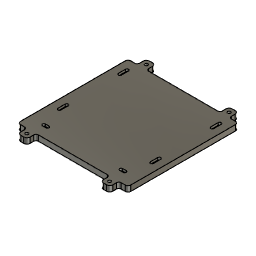
base_mount (Autodesk Fusion 360 design; units mm, degrees)
Autodesk Fusion 360 part; units mm, degrees
sketch "Sketch1" plane through (0, 0, 0) normal (0, 0, 1) x (1, 0, 0)
  line L0 (60, -60) -> (-60, -60)
  line L1 (-60, -60) -> (-60, 60)
  line L2 (-60, 60) -> (60, 60)
  line L3 (60, 60) -> (60, -60)
  line L4 (60, -60) -> (-60, 60) construction
  line L5 (-60, -60) -> (60, 60) construction
  dimension "d4" = 120
  dimension "d5" = 120
  constraint perpendicular L0 L1
  constraint parallel L0 L2
  constraint parallel L1 L3
  constraint horizontal L0
  constraint coincident L4 origin
  constraint coincident L5 origin
  measures "d4" distance of L1.end L2.end
  measures "d5" distance of L0.end L1.end
extrude "Extrude1" add sketch "Sketch1" along normal blind 6
sketch "Sketch2" plane through (0, 0, 0) normal (0, 0, -1) x (1, 0, 0)
  line L0 (-60, -60) -> (60, -60)
  line L1 (60, -60) -> (60, 60)
  line L2 (60, 60) -> (-60, 60)
  line L3 (-60, 60) -> (-60, -60)
  line L4 (-44, 44.625) -> (-40, 44.625)
  arc A0 (-40, 44.625) -> (-40, 50.375) centre (-40, 47.5) ccw
  line L5 (-40, 50.375) -> (-44, 50.375)
  arc A1 (-44, 50.375) -> (-44, 44.625) centre (-44, 47.5) ccw
  line L6 (-44, 47.5) -> (-40, 47.5) construction
  point P0 (-42, 47.5)
  dimension "d14" = 5.75
  dimension "d15" = 4
  dimension "d16" = 12.5
  dimension "d17" = 18
  constraint tangent L4 A0
  constraint tangent A0 L5
  constraint parallel L4 L5
  constraint tangent L5 A1
  constraint tangent L4 A1
  constraint horizontal L6
  constraint midpoint L6 P0
  measures "d14" diameter of A0
  measures "d15" distance of A1.centre A0.centre
  measures "d16" distance of L2 P0
  measures "d17" distance of L3 P0
extrude "Extrude2" cut sketch "Sketch2" against normal blind 3.5 contours L4 A0 L5 A1
sketch "Sketch3" plane through (0, 0, 3.5) normal (0, 0, -1) x (1, 0, 0)
  arc A0 (-44, 50.375) -> (-44, 44.625) centre (-44, 47.5) ccw
  line L0 (-44, 44.625) -> (-40, 44.625)
  arc A1 (-40, 44.625) -> (-40, 50.375) centre (-40, 47.5) ccw
  line L1 (-40, 50.375) -> (-44, 50.375)
  line L2 (-44, 45.875) -> (-40, 45.875)
  arc A2 (-40, 45.875) -> (-40, 49.125) centre (-40, 47.5) ccw
  line L3 (-40, 49.125) -> (-44, 49.125)
  arc A3 (-44, 49.125) -> (-44, 45.875) centre (-44, 47.5) ccw
  line L4 (-44, 47.5) -> (-40, 47.5) construction
  line L5 (60, 60) -> (-60, 60)
  line L6 (-60, 60) -> (-60, -60)
  point P0 (-42, 47.5)
  dimension "d20" = 3.25
  dimension "d21" = 4
  dimension "d22" = 12.5
  dimension "d23" = 18
  constraint tangent L2 A2
  constraint tangent A2 L3
  constraint parallel L2 L3
  constraint tangent L3 A3
  constraint tangent L2 A3
  constraint parallel L0 L4
  constraint midpoint L4 P0
  measures "d20" diameter of A2
  measures "d21" distance of A0.centre A1.centre
  measures "d22" distance of P0 L5
  measures "d23" distance of P0 L6
extrude "Extrude3" cut sketch "Sketch3" against normal up to surface (2.5 mm away) contours L2 A2 L3 A3
mirror "Mirror1" about plane through (0, 0, 0) normal (1, 0, 0) of "Extrude2", "Extrude3"
sketch "Sketch4" plane through (0, 0, 0) normal (0, 0, -1) x (1, 0, 0)
  line L0 (44, 44.625) -> (40, 44.625)
  arc A0 (40, 50.375) -> (40, 44.625) centre (40, 47.5) ccw
  line L1 (40, 50.375) -> (44, 50.375)
  arc A1 (44, 44.625) -> (44, 50.375) centre (44, 47.5) ccw
  line L2 (-40, 44.625) -> (-44, 44.625)
  arc A2 (-44, 50.375) -> (-44, 44.625) centre (-44, 47.5) ccw
  line L3 (-44, 50.375) -> (-40, 50.375)
  arc A3 (-40, 44.625) -> (-40, 50.375) centre (-40, 47.5) ccw
  line L4 (-60, -60) -> (60, -60)
  line L5 (60, -60) -> (60, 60)
  line L6 (60, 60) -> (-60, 60)
  line L7 (-60, 60) -> (-60, -60)
  line L8 (60, -60) -> (-60, -60) construction
  line L9 (-60, -60) -> (-60, 35) construction
  line L10 (-60, 35) -> (60, 35) construction
  line L11 (60, 35) -> (60, -60) construction
  line L12 (0, 35) -> (0, -60) construction
  line L13 (60, -12.5) -> (-60, -12.5) construction
  line L14 (-50.35, -45.35) -> (50.35, -45.35) construction
  line L15 (50.35, -45.35) -> (50.35, 20.35) construction
  line L16 (50.35, 20.35) -> (-50.35, 20.35) construction
  line L17 (-50.35, 20.35) -> (-50.35, -45.35) construction
  line L18 (-50.35, -45.35) -> (50.35, 20.35) construction
  line L19 (50.35, -45.35) -> (-50.35, 20.35) construction
  line L20 (47.475, 24.35) -> (47.475, 16.35)
  arc A4 (47.475, 16.35) -> (53.225, 16.35) centre (50.35, 16.35) ccw
  line L21 (53.225, 16.35) -> (53.225, 24.35)
  arc A5 (53.225, 24.35) -> (47.475, 24.35) centre (50.35, 24.35) ccw
  line L22 (50.35, 24.35) -> (50.35, 16.35) construction
  line L23 (51.975, 16.35) -> (51.975, 24.35)
  arc A6 (51.975, 24.35) -> (48.725, 24.35) centre (50.35, 24.35) ccw
  line L24 (48.725, 24.35) -> (48.725, 16.35)
  arc A7 (48.725, 16.35) -> (51.975, 16.35) centre (50.35, 16.35) ccw
  line L25 (50.35, 16.35) -> (50.35, 24.35) construction
  point P0 (0, -12.5)
  point P1 (50.35, 20.35)
  point P2 (50.35, 20.35)
  dimension "d29" = 95
  dimension "d30" = 65.7
  dimension "d31" = 100.7
  dimension "d36" = 5.75
  dimension "d37" = 8
  dimension "d38" = 3.25
  dimension "d39" = 8
  constraint horizontal L8
  constraint vertical L9
  constraint horizontal L10
  constraint vertical L11
  constraint coincident L4.end L5.start
  constraint midpoint L10 L12.start
  constraint midpoint L8 L12.end
  constraint midpoint L11 L13.start
  constraint midpoint L9 L13.end
  constraint perpendicular L14 L15
  constraint parallel L14 L16
  constraint parallel L15 L17
  constraint horizontal L14
  constraint coincident L18 P0
  constraint coincident L19 P0
  constraint midpoint L13 P0
  constraint tangent L20 A4
  constraint tangent A4 L21
  constraint parallel L20 L21
  constraint tangent L21 A5
  constraint tangent L20 A5
  constraint coincident L15 A4.centre
  constraint perpendicular L16 L22
  constraint coincident P2 P1
  constraint midpoint L22 P2
  constraint tangent L23 A6
  constraint tangent A6 L24
  constraint parallel L23 L24
  constraint tangent L24 A7
  constraint tangent L23 A7
  constraint coincident L22 A5.centre
  constraint perpendicular L16 L25
  constraint midpoint L25 P2
  measures "d29" distance of L4.end L10.end
  measures "d30" distance of L14.end P2
  measures "d31" distance of P2 L16.end
  measures "d36" diameter of A4
  measures "d37" distance of A5.centre A4.centre
  measures "d38" diameter of A6
  measures "d39" distance of A4.centre A5.centre
extrude "Extrude4" cut sketch "Sketch4" against normal blind 3.5 contours L20 A4 L21 A5
extrude "Extrude5" cut sketch "Sketch4" against normal up to surface (6 mm away) contours L23 A6 L24 A7
pattern_linear "R-Pattern1" count 2 spacing 100.7 along (-1, 0, 0) count 2 spacing 65.7 along (0, 1, 0) of "Extrude4", "Extrude5"
sketch "Sketch5" plane through (0, 0, 0) normal (0, 0, -1) x (1, 0, 0)
  line L0 (47.475, -49.35) -> (47.475, -41.35)
  arc A0 (53.225, -41.35) -> (47.475, -41.35) centre (50.35, -41.35) ccw
  line L1 (53.225, -41.35) -> (53.225, -49.35)
  arc A1 (47.475, -49.35) -> (53.225, -49.35) centre (50.35, -49.35) ccw
  line L2 (47.475, 16.35) -> (47.475, 24.35)
  arc A2 (53.225, 24.35) -> (47.475, 24.35) centre (50.35, 24.35) ccw
  line L3 (53.225, 24.35) -> (53.225, 16.35)
  arc A3 (47.475, 16.35) -> (53.225, 16.35) centre (50.35, 16.35) ccw
  line L4 (44, 44.625) -> (40, 44.625)
  arc A4 (40, 50.375) -> (40, 44.625) centre (40, 47.5) ccw
  line L5 (40, 50.375) -> (44, 50.375)
  arc A5 (44, 44.625) -> (44, 50.375) centre (44, 47.5) ccw
  line L6 (-40, 44.625) -> (-44, 44.625)
  arc A6 (-44, 50.375) -> (-44, 44.625) centre (-44, 47.5) ccw
  line L7 (-44, 50.375) -> (-40, 50.375)
  arc A7 (-40, 44.625) -> (-40, 50.375) centre (-40, 47.5) ccw
  line L8 (-60, -60) -> (60, -60)
  line L9 (60, -60) -> (60, 60)
  line L10 (60, 60) -> (-60, 60)
  line L11 (-60, 60) -> (-60, -60)
  line L12 (-53.225, 16.35) -> (-53.225, 24.35)
  arc A8 (-47.475, 24.35) -> (-53.225, 24.35) centre (-50.35, 24.35) ccw
  line L13 (-47.475, 24.35) -> (-47.475, 16.35)
  arc A9 (-53.225, 16.35) -> (-47.475, 16.35) centre (-50.35, 16.35) ccw
  line L14 (-53.225, -49.35) -> (-53.225, -41.35)
  arc A10 (-47.475, -41.35) -> (-53.225, -41.35) centre (-50.35, -41.35) ccw
  line L15 (-47.475, -41.35) -> (-47.475, -49.35)
  arc A11 (-53.225, -49.35) -> (-47.475, -49.35) centre (-50.35, -49.35) ccw
  line L16 (49.25, 50) -> (-49.25, 50) construction
  line L17 (-49.25, 50) -> (-49.25, -50) construction
  line L18 (-49.25, -50) -> (49.25, -50) construction
  line L19 (49.25, -50) -> (49.25, 50) construction
  line L20 (49.25, 50) -> (-49.25, -50) construction
  line L21 (-49.25, 50) -> (49.25, -50) construction
  line L22 (7.5, 50.4) -> (-2.5, 50.4)
  line L23 (-2.5, 50.4) -> (-2.5, 52.4)
  line L24 (-2.5, 52.4) -> (7.5, 52.4)
  line L25 (7.5, 52.4) -> (7.5, 50.4)
  line L26 (7.5, 50.4) -> (-2.5, 52.4) construction
  line L27 (-2.5, 50.4) -> (7.5, 52.4) construction
  line L28 (-51.65, 5.3028) -> (-49.65, 5.3028)
  line L29 (-49.65, 5.3028) -> (-49.65, -4.6972)
  line L30 (-49.65, -4.6972) -> (-51.65, -4.6972)
  line L31 (-51.65, -4.6972) -> (-51.65, 5.3028)
  line L32 (-51.65, 5.3028) -> (-49.65, -4.6972) construction
  line L33 (-49.65, 5.3028) -> (-51.65, -4.6972) construction
  line L34 (51.65, -5) -> (49.65, -5)
  line L35 (49.65, -5) -> (49.65, 5)
  line L36 (49.65, 5) -> (51.65, 5)
  line L37 (51.65, 5) -> (51.65, -5)
  line L38 (51.65, -5) -> (49.65, 5) construction
  line L39 (49.65, -5) -> (51.65, 5) construction
  line L40 (5.2107, -52.4) -> (-4.7893, -52.4)
  line L41 (-4.7893, -52.4) -> (-4.7893, -50.4)
  line L42 (-4.7893, -50.4) -> (5.2107, -50.4)
  line L43 (5.2107, -50.4) -> (5.2107, -52.4)
  line L44 (5.2107, -52.4) -> (-4.7893, -50.4) construction
  line L45 (-4.7893, -52.4) -> (5.2107, -50.4) construction
  point P0 (2.5, 51.4)
  point P1 (-50.65, 0.3028)
  point P2 (50.65, 0)
  point P3 (0.2107, -51.4)
  dimension "d50" = 100
  dimension "d51" = 98.5
  dimension "d56" = 10
  dimension "d57" = 2
  dimension "d58" = 0.4
  dimension "d59" = 10
  dimension "d60" = 2
  dimension "d61" = 0.4
  dimension "d62" = 2
  dimension "d63" = 10
  dimension "d64" = 0.4
  dimension "d65" = 10
  dimension "d66" = 2
  dimension "d67" = 0.4
  constraint perpendicular L16 L17
  constraint parallel L16 L18
  constraint parallel L17 L19
  constraint horizontal L16
  constraint coincident L20 origin
  constraint coincident L21 origin
  constraint perpendicular L22 L23
  constraint parallel L22 L24
  constraint parallel L23 L25
  constraint horizontal L22
  constraint coincident L26 P0
  constraint coincident L27 P0
  constraint perpendicular L28 L29
  constraint parallel L28 L30
  constraint parallel L29 L31
  constraint horizontal L28
  constraint coincident L32 P1
  constraint coincident L33 P1
  constraint perpendicular L34 L35
  constraint parallel L34 L36
  constraint parallel L35 L37
  constraint horizontal L34
  constraint coincident L38 P2
  constraint coincident L39 P2
  constraint perpendicular L40 L41
  constraint parallel L40 L42
  constraint parallel L41 L43
  constraint horizontal L40
  constraint coincident L44 P3
  constraint coincident L45 P3
  measures "d50" distance of L16.end L17.end
  measures "d51" distance of L17.end L18.end
  measures "d56" distance of L23.end L24.end
  measures "d57" distance of L22.end L23.end
  measures "d58" distance of L16 L22
  measures "d59" distance of L28.end L29.end
  measures "d60" distance of L29.end L30.end
  measures "d61" distance of L17 L29
  measures "d62" distance of L35.end L36.end
  measures "d63" distance of L34.end L35.end
  measures "d64" distance of L19 L35
  measures "d65" distance of L41.end L42.end
  measures "d66" distance of L40.end L41.end
  measures "d67" distance of L18 L42
extrude "Extrude6" add sketch "Sketch5" along normal blind 3.5 contours L22 L23 L24 L25 | L28 L29 L30 L31 | L34 L35 L36 L37 | L40 L41 L42 L43
sketch "Sketch6" plane through (0, 0, 6) normal (0, 0, 1) x (-1, 0, 0)
  line L0 (51.975, -41.35) -> (51.975, -49.35)
  arc A0 (48.725, -49.35) -> (51.975, -49.35) centre (50.35, -49.35) ccw
  line L1 (48.725, -49.35) -> (48.725, -41.35)
  arc A1 (51.975, -41.35) -> (48.725, -41.35) centre (50.35, -41.35) ccw
  line L2 (-48.725, -41.35) -> (-48.725, -49.35)
  arc A2 (-51.975, -49.35) -> (-48.725, -49.35) centre (-50.35, -49.35) ccw
  line L3 (-51.975, -49.35) -> (-51.975, -41.35)
  arc A3 (-48.725, -41.35) -> (-51.975, -41.35) centre (-50.35, -41.35) ccw
  line L4 (51.975, 24.35) -> (51.975, 16.35)
  arc A4 (48.725, 16.35) -> (51.975, 16.35) centre (50.35, 16.35) ccw
  line L5 (48.725, 16.35) -> (48.725, 24.35)
  arc A5 (51.975, 24.35) -> (48.725, 24.35) centre (50.35, 24.35) ccw
  line L6 (-48.725, 24.35) -> (-48.725, 16.35)
  arc A6 (-51.975, 16.35) -> (-48.725, 16.35) centre (-50.35, 16.35) ccw
  line L7 (-51.975, 16.35) -> (-51.975, 24.35)
  arc A7 (-48.725, 24.35) -> (-51.975, 24.35) centre (-50.35, 24.35) ccw
  line L8 (-40, 45.875) -> (-44, 45.875)
  arc A8 (-44, 49.125) -> (-44, 45.875) centre (-44, 47.5) ccw
  line L9 (-44, 49.125) -> (-40, 49.125)
  arc A9 (-40, 45.875) -> (-40, 49.125) centre (-40, 47.5) ccw
  line L10 (40, 49.125) -> (44, 49.125)
  arc A10 (44, 45.875) -> (44, 49.125) centre (44, 47.5) ccw
  line L11 (44, 45.875) -> (40, 45.875)
  arc A11 (40, 49.125) -> (40, 45.875) centre (40, 47.5) ccw
  line L12 (-60, -60) -> (60, -60)
  line L13 (60, -60) -> (60, 60)
  line L14 (60, 60) -> (-60, 60)
  line L15 (-60, 60) -> (-60, -60)
sketch "Sketch7" plane through (0, 0, 6) normal (0, 0, 1) x (-1, 0, 0)
  line L0 (51.975, -41.35) -> (51.975, -49.35)
  arc A0 (48.725, -49.35) -> (51.975, -49.35) centre (50.35, -49.35) ccw
  line L1 (48.725, -49.35) -> (48.725, -41.35)
  arc A1 (51.975, -41.35) -> (48.725, -41.35) centre (50.35, -41.35) ccw
  line L2 (-48.725, -41.35) -> (-48.725, -49.35)
  arc A2 (-51.975, -49.35) -> (-48.725, -49.35) centre (-50.35, -49.35) ccw
  line L3 (-51.975, -49.35) -> (-51.975, -41.35)
  arc A3 (-48.725, -41.35) -> (-51.975, -41.35) centre (-50.35, -41.35) ccw
  line L4 (51.975, 24.35) -> (51.975, 16.35)
  arc A4 (48.725, 16.35) -> (51.975, 16.35) centre (50.35, 16.35) ccw
  line L5 (48.725, 16.35) -> (48.725, 24.35)
  arc A5 (51.975, 24.35) -> (48.725, 24.35) centre (50.35, 24.35) ccw
  line L6 (-48.725, 24.35) -> (-48.725, 16.35)
  arc A6 (-51.975, 16.35) -> (-48.725, 16.35) centre (-50.35, 16.35) ccw
  line L7 (-51.975, 16.35) -> (-51.975, 24.35)
  arc A7 (-48.725, 24.35) -> (-51.975, 24.35) centre (-50.35, 24.35) ccw
  line L8 (-40, 45.875) -> (-44, 45.875)
  arc A8 (-44, 49.125) -> (-44, 45.875) centre (-44, 47.5) ccw
  line L9 (-44, 49.125) -> (-40, 49.125)
  arc A9 (-40, 45.875) -> (-40, 49.125) centre (-40, 47.5) ccw
  line L10 (40, 49.125) -> (44, 49.125)
  arc A10 (44, 45.875) -> (44, 49.125) centre (44, 47.5) ccw
  line L11 (44, 45.875) -> (40, 45.875)
  arc A11 (40, 49.125) -> (40, 45.875) centre (40, 47.5) ccw
  line L12 (-60, -60) -> (60, -60)
  line L13 (60, -60) -> (60, 60)
  line L14 (60, 60) -> (-60, 60)
  line L15 (-60, 60) -> (-60, -60)
  line L16 (50, 60) -> (40, 60)
  line L17 (40, 60) -> (40, 70)
  line L18 (40, 70) -> (50, 70)
  line L19 (50, 70) -> (50, 60)
  circle A12 centre (45, 65) radius 1.625
  line L20 (0, -80) -> (0, 80) construction
  line L21 (75, 0) -> (-75, 0) construction
  circle A13 centre (-45, 65) radius 1.625
  line L22 (-50, 60) -> (-40, 60)
  line L23 (-40, 70) -> (-50, 70)
  line L24 (-40, 60) -> (-40, 70)
  line L25 (-50, 70) -> (-50, 60)
  line L26 (40, -70) -> (50, -70)
  line L27 (0, 80) -> (0, -80) construction
  line L28 (-40, -70) -> (-50, -70)
  line L29 (50, -60) -> (40, -60)
  circle A14 centre (-45, -65) radius 1.625
  line L30 (40, -60) -> (40, -70)
  circle A15 centre (45, -65) radius 1.625
  line L31 (50, -70) -> (50, -60)
  line L32 (-40, -60) -> (-40, -70)
  line L33 (-50, -70) -> (-50, -60)
  dimension "d78" = 10
  dimension "d79" = 10
  dimension "d80" = 10
  dimension "d81" = 3.25
  dimension "d83" = 5
  dimension "d84" = 5
  constraint horizontal L16
  constraint vertical L17
  constraint horizontal L18
  constraint vertical L19
  constraint coincident L14 L16.start
  constraint parallel L15 L20
  constraint perpendicular L15 L21
  constraint symmetric L16.start L20 L22.start
  constraint symmetric L16.end L20 L22.end
  constraint symmetric L17.end L20 L23.start
  constraint symmetric L18.end L20 L23.end
  constraint symmetric A12 L20 A13
  constraint symmetric L16.start L21 L29.start
  constraint symmetric L16.end L21 L29.end
  constraint symmetric L17.end L21 L26.start
  constraint symmetric L18.end L21 L26.end
  constraint symmetric A12 L21 A15
  constraint symmetric L20.start L21 L20.end
  constraint symmetric L20.end L21 L20.start
  constraint symmetric L21 L22.end L32.start
  constraint symmetric L21 L22.start L33.end
  constraint symmetric L21 L23.end L28.end
  constraint symmetric L21 L23.start L28.start
  constraint symmetric L21 A13 A14
  measures "d78" distance of L16.start L16.end
  measures "d79" distance of L16.start L18.end
  measures "d80" distance of L13 L19
  measures "d81" diameter of A12
  measures "d83" distance of L18 A12.centre
  measures "d84" distance of L17 A12.centre
extrude "Extrude7" add sketch "Sketch7" against normal up to surface (6 mm away) contours L12 L28 L32 L33 | L14 L22 L23 L24 L25 | L12 L26 L29 L30 L31 | L14 L16 L17 L18 L19
fillet "Fillet1" radius 3.5 2 edges at (-50, -70, 3) (-40, -70, 3)
fillet "Fillet2" radius 3.5 2 edges at (40, -70, 3) (50, -70, 3)
fillet "Fillet3" radius 3.5 2 edges at (-40, 70, 3) (-50, 70, 3)
fillet "Fillet4" radius 3.5 2 edges at (40, 70, 3) (50, 70, 3)
fillet "Fillet5" radius 2.5 8 edges at (50, 60, 3) (40, 60, 3) (-40, 60, 3) (-50, 60, 3) (-50, -60, 3) (50, -60, 3) (-40, -60, 3) (40, -60, 3)
fillet "Fillet6" radius 3 4 edges at (-60, 60, 3) (-60, -60, 3) (60, -60, 3) (60, 60, 3)
move_face "MoveFace1" by (-8.35, 0, 0) 10 faces at (-51.65, 1.3639, -1.1667) (-50.3167, 4.6972, -1.1667) (-50.9833, -1.9695, -3.5) (-50.9833, -5.3028, -1.1667) (-49.65, -1.9695, -1.1667) (50.3167, -5, -1.1667) (50.9833, 1.6667, -3.5) (51.65, -1.6667, -1.1667) (50.9833, 5, -1.1667) (49.65, 1.6667, -1.1667)
move_face "MoveFace2" by (-0.2, 0, 0) 5 faces at (41.3, 1.6667, -1.1667) (42.6333, 5, -1.1667) (42.6333, 1.6667, -3.5) (42.6333, -5, -1.1667) (43.3, -1.6667, -1.1667)
equation "base_width = 120 mm"
equation "base_length = 120 mm"
equation "base_thickness = 6 mm"
equation "d4 = base_width"
equation "d5 = base_length"
equation "d6 = base_thickness"
equation "fan_mount_hole_long_edge_offset = 18 mm"
equation "fan_bottom_mount_hole_head_countersink = 3.5 mm"
equation "fan_bottom_mount_hole_diameter = 3.25 mm"
equation "fan_bottom_mount_hole_head_diameter = 5.75 mm"
equation "fan_bottom_mount_hole_slot_length = 4 mm"
equation "fan_mount_hole_short_edge_offset = 12.5 mm"
equation "d14 = fan_bottom_mount_hole_head_diameter"
equation "d15 = fan_bottom_mount_hole_slot_length"
equation "d16 = fan_mount_hole_short_edge_offset"
equation "d17 = fan_mount_hole_long_edge_offset"
equation "d18 = -fan_bottom_mount_hole_head_countersink"
equation "d20 = fan_bottom_mount_hole_diameter"
equation "d21 = fan_bottom_mount_hole_slot_length"
equation "d22 = fan_mount_hole_short_edge_offset"
equation "d23 = fan_mount_hole_long_edge_offset"
equation "pi_mount_width = 65.7 mm"
equation "pi_mount_length = 100.7 mm"
equation "d30 = pi_mount_width"
equation "d31 = pi_mount_length"
equation "pi_bottom_mount_hole_diameter = 3.25 mm"
equation "pi_bottom_mount_hole_head_countersink = 3.5 mm"
equation "pi_bottom_mount_hole_head_diameter = 5.75 mm"
equation "pi_bottom_mount_hole_slot_length = 8 mm"
equation "d36 = pi_bottom_mount_hole_head_diameter"
equation "d37 = pi_bottom_mount_hole_slot_length"
equation "d38 = pi_bottom_mount_hole_diameter"
equation "d39 = pi_bottom_mount_hole_slot_length"
equation "d40 = -pi_bottom_mount_hole_head_countersink"
equation "d46 = pi_mount_length"
equation "d47 = pi_mount_width"
equation "switch_width = 100 mm"
equation "switch_length = 98.5 mm"
equation "d50 = switch_width"
equation "d51 = switch_length"
equation "switch_lateral_support_length = 10 mm"
equation "switch_lateral_support_offset = 0.4 mm"
equation "switch_lateral_support_thickness = 3.5 mm"
equation "switch_lateral_support_width = 2 mm"
equation "d56 = switch_lateral_support_length"
equation "d57 = switch_lateral_support_width"
equation "d58 = switch_lateral_support_offset"
equation "d59 = switch_lateral_support_length"
equation "d60 = switch_lateral_support_width"
equation "d61 = switch_lateral_support_offset"
equation "d62 = switch_lateral_support_width"
equation "d63 = switch_lateral_support_length"
equation "d64 = switch_lateral_support_offset"
equation "d65 = switch_lateral_support_length"
equation "d66 = switch_lateral_support_width"
equation "d67 = switch_lateral_support_offset"
equation "d68 = switch_lateral_support_thickness"
equation "base_bracket_width = 10 mm"
equation "base_bracket_edge_offset = 10 mm"
equation "base_bracket_hole_diameter = 3.25 mm"
equation "base_bracket_length = 10 mm"
equation "base_bracket_hole_edge_offset = 5 mm"
equation "d78 = base_bracket_width"
equation "d79 = base_bracket_length"
equation "d80 = base_bracket_edge_offset"
equation "d81 = base_bracket_hole_diameter"
equation "base_bracket_length_edge_offset = 5 mm"
equation "d83 = base_bracket_length_edge_offset"
equation "d84 = base_bracket_width / 2"
equation "base_bracket_outer_fillet = 3.5 mm"
equation "base_bracket_inner_fillet = 2.5 mm"
equation "d89 = base_bracket_outer_fillet"
equation "d90 = base_bracket_outer_fillet"
equation "d91 = base_bracket_outer_fillet"
equation "d92 = base_bracket_outer_fillet"
equation "d93 = base_bracket_inner_fillet"
equation "base_edge_fillet = 3 mm"
equation "d95 = base_edge_fillet"
